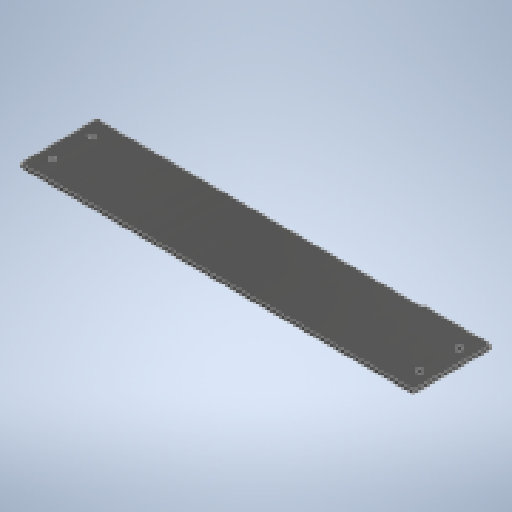
# Autodesk Inventor part: 2309HCMUTE-CDT23_TAM-GA
Saved by Autodesk Inventor 2023 (Build 270158000, 158)
## iProperties
Created: 2023-10-13
Part Number: 2309HCMUTE-CDT23_TAM-GA
Material: PMMA Plastic
Document SubType Name: Modeling
Designer: havie
Density: 1.188 g/cm^3
Appearance: Dark Gray
Author: havie
Autodesk Inventor part; units mm, degrees
ref_plane "YZ Plane" through (0, 0, 0) normal (1, 0, 0) x (0, 1, 0)
ref_plane "XZ Plane" through (0, 0, 0) normal (0, 1, 0) x (-1, 0, 0)
ref_plane "XY Plane" through (0, 0, 0) normal (0, 0, 1) x (1, 0, 0)
sketch "Sketch1" plane through (0, 0, 0) normal (0, 1, 0) x (-1, 0, 0)
  line L0 (125, 30) -> (-125, 30)
  line L1 (-125, 30) -> (-125, -30)
  line L2 (-125, -30) -> (125, -30)
  line L3 (125, -30) -> (125, 30)
  line L4 (125, 30) -> (-125, -30) construction
  line L5 (-125, 30) -> (125, -30) construction
  point P0 (0, 0)
  dimension "d0" = 250
  dimension "d1" = 60
  constraints: 12 end point, 2 midpoint, 2 parallel, 1 horizontal, 1 perpendicular
  measures "d0" distance of L1.end L2.end
  measures "d1" distance of L2.end L0.start
extrude "Extrusion1" add sketch "Sketch1" along normal mid plane 3
sketch "Sketch2" plane through (0, -1.5, 0) normal (0, -1, 0) x (1, 0, 0)
  line L0 (125, -30) -> (125, 30) projected
  line L1 (125, 30) -> (-125, 30) projected
  line L2 (-125, 30) -> (-125, -30) projected
  point P0 (0, 0)
  point P1 (113.5, 15)
  point P2 (113.5, -15)
  point P3 (-113.5, 15)
  point P4 (-113.5, -15)
  dimension "d9" = 11.5
  dimension "d10" = 15
  dimension "d11" = 30
  dimension "d12" = 11.5
  constraints: 2 horizontal alignment, 2 vertical alignment
  measures "d9" distance from line of point (113.5, 15) L0
  measures "d10" distance from line of L1 point (113.5, 15)
  measures "d11" distance of point (113.5, -15) point (113.5, 15)
  measures "d12" distance from line of L2 point (-113.5, 15)
hole "Hole1" at (113.5, -1.5, 15) at (113.5, -1.5, -15) at (-113.5, -1.5, 15) at (-113.5, -1.5, -15) direction (0, 1, 0) diameter 4.4587 depth 12.8 tip angle 118 thread size "M5x0.5" class "6H" standard "ISO Metric profile"
sketch "Sketch3" plane through (0, 1.5, 0) normal (0, 1, 0) x (1, 0, 0)
  line L0 (125, 30.7071) -> (125, 28.5858) projected
  line L1 (125, 30) -> (-125, 30) projected
  line L2 (-125, 30) -> (-125, -30) projected
  line L3 (125, 30) -> (-125, 30)
  line L4 (-125, 30) -> (-125, 25)
  line L5 (-125, 25) -> (125, 25)
  line L6 (125, 25) -> (125, 30)
  point P0 (0, 0)
  dimension "d20" = 5
  constraints: 8 end point, 3 point on line, 2 parallel, 1 horizontal, 1 perpendicular
  measures "d20" distance between parallel lines of L1 L5
extrude "Extrusion2" cut sketch "Sketch3" against normal blind 3
body "Solid1"
